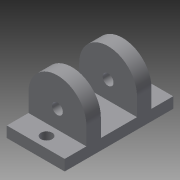
# Autodesk Inventor part: clip_hinge
Saved by Autodesk Inventor 2015 (Build 190159000, 159)
## iProperties
Created: 2017-10-02
Part Number: clip_hinge
Material: Generic
Document SubType Name: Modeling
Designer: Anshul
Density: 1 g/cm^3
Appearance: Default
Author: Anshul
Autodesk Inventor part; units mm, degrees
ref_plane "YZ Plane" through (0, 0, 0) normal (1, 0, 0) x (0, 1, 0)
ref_plane "XZ Plane" through (0, 0, 0) normal (0, 1, 0) x (-1, 0, 0)
ref_plane "XY Plane" through (0, 0, 0) normal (0, 0, 1) x (1, 0, 0)
sketch "Sketch1" plane through (0, 0, 0) normal (0, 1, 0) x (-1, 0, 0)
  line L0 (0, 0) -> (0, -30)
  line L1 (0, -30) -> (16, -30)
  line L2 (16, -30) -> (16, 0)
  line L3 (16, 0) -> (0, 0)
  line L4 (8, 0) -> (8, -3)
  line L5 (8, -30) -> (8, -27)
  circle A0 centre (8, -3) radius 1.55
  circle A1 centre (8, -27) radius 1.55
  line L6 (8, -24) -> (0, -24)
  line L7 (8, -24) -> (16, -24)
  line L8 (8, -6) -> (0, -6)
  line L9 (8, -6) -> (16, -6)
  line L10 (16, -6) -> (16, -10)
  line L11 (16, -10) -> (0, -10)
  line L12 (16, -24) -> (16, -20)
  line L13 (16, -20) -> (0, -20)
  dimension "d0" = 30
  dimension "d1" = 16
  dimension "d2" = 3
  dimension "d3" = 3
  dimension "d4" = 3.1
  dimension "d5" = 3.1
  dimension "d6" = 3
  dimension "d7" = 3
  dimension "d8" = 4
  dimension "d9" = 4
  constraints: 28 end point, 11 point on line, 7 perpendicular, 2 centre point, 2 coincident, 2 midpoint, 2 vertical
  measures "d0" distance of L0.start L0.end
  measures "d1" distance of L0.end L1.end
  measures "d2" distance of L4.start L4.end
  measures "d3" distance of L5.start L5.end
  measures "d4" diameter of A0
  measures "d5" diameter of A1
  measures "d6" distance of A0.centre L8.start
  measures "d7" distance of A1.centre L6.start
  measures "d8" distance of L9.end L10.end
  measures "d9" distance of L7.end L12.end
extrude "Extrusion1" add sketch "Sketch1" against normal blind 3
extrude "Extrusion2" add sketch "Sketch1" along normal blind 5 contours L8 L9 L2 L11 L0 | L13 L2 L7 L6 L0
sketch "Sketch2" plane through (-16, 0, -6) normal (0, 0, 1) x (1, 0, 0)
  line L0 (16, 5) -> (0, 5) projected
  arc A0 (16, 5) -> (0, 5) centre (8, 5) ccw
  line L1 (0, 5) -> (16, 5)
  line L2 (16, 0) -> (16, 5) projected
  arc A1 (9.5, 5) -> (6.5, 5) centre (8, 5) ccw
  circle A2 centre (8, 5) radius 1.5
  dimension "d14" = 3
  constraints: 4 point on circle, 3 end point, 2 centre point, 2 coincident, 2 point on line, 1 horizontal alignment, 1 midpoint, 1 perpendicular, 2 other
  measures "d14" diameter of A1
extrude "Extrusion3" add sketch "Sketch2" against normal blind 4 contours L0 A1 A0
sketch "Sketch3" plane through (0, 0, -24) normal (0, 0, -1) x (-1, 0, 0)
  line L0 (6.5, 5) -> (9.5, 5) projected
  arc A0 (9.5, 5) -> (6.5, 5) centre (8, 5) ccw
  arc A1 (16, 5) -> (0, 5) centre (8, 5) ccw
  line L1 (0, 5) -> (16, 5)
  point P0 (0, 0)
  constraints: 5 point on circle, 2 centre point, 2 end point, 2 point on line, 1 coincident, 1 horizontal, 1 midpoint
extrude "Extrusion4" add sketch "Sketch3" against normal blind 4 contours L1 A1 A0
extrude "Extrusion5" cut sketch "Sketch2" against normal blind 30 contours A2 L0 | L0 A1
body "Solid1"
